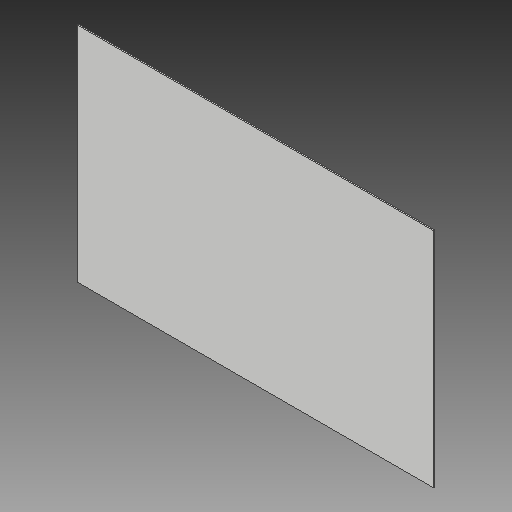
# Autodesk Inventor part: ApoioBocalInferior_
Saved by Autodesk Inventor 2018 (Build 220112000, 112)
## iProperties
Created: 2018-07-25
Part Number: ApoioBocalInferior_
Material: Genérico
Document SubType Name: Chapa de metal
Designer: Usuario
Density: 1 g/cm^3
Sheet Metal Rule: Padrão_mm
Appearance: Padrão
Mass: 6.48 g
Surface Area: 261.54 cm^2
Volume: 6.48 cm^3
Author: Usuario
Autodesk Inventor part; units mm, degrees
ref_plane "YZ Plane" through (0, 0, 0) normal (1, 0, 0) x (0, 1, 0)
ref_plane "XZ Plane" through (0, 0, 0) normal (0, 1, 0) x (-1, 0, 0)
ref_plane "XY Plane" through (0, 0, 0) normal (0, 0, 1) x (1, 0, 0)
sketch "Esboço1" plane through (0, 0, 0) normal (0, 0, 1) x (1, 0, 0)
  line L0 (-6, 80.4039) -> (-150, 80.4039)
  line L1 (-150, 80.4039) -> (-150, 170.4039)
  line L2 (-150, 170.4039) -> (-6, 170.4039)
  line L3 (-6, 170.4039) -> (-6, 80.4039)
  point P0 (0, 0)
  dimension "d0" = 144
  dimension "d1" = 90
  measures "d0" distance of L1.end L2.end
  measures "d1" distance of L0.end L1.end
extrude "Placa1" add sketch "Esboço1" along normal blind 0.5
equation "\"Raio_vergadura\" = Espessura"
equation "\"Largura_alívio_de_vergadura\" = Espessura"
equation "\"Profundidade_alívio_de_vergadura\" = 0.5 * Espessura"
equation "\"Tamanho_alívio_de_dobra\" = 4 * Espessura"
equation "\"Remanescente_mínimo\" = 2 * Espessura"
equation "\"Raiodetransição\" = Raio_vergadura"
equation "\"Tamanho_de_raio_de_Jacobi\" = Raio_vergadura"
equation "\"TamanhoFolga\" = Espessura"
